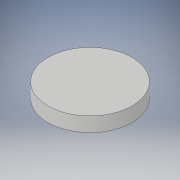
# Autodesk Inventor part: Speaker
Saved by Autodesk Inventor 2018 (Build 220112000, 112)
## iProperties
Created: 2017-05-31
Part Number: Speaker
Material: Generic
Document SubType Name: Modeling
Designer: Rishi
Density: 1 g/cm^3
Appearance: Default
Author: Rishi
Autodesk Inventor part; units mm, degrees
ref_plane "YZ Plane" through (0, 0, 0) normal (1, 0, 0) x (0, 1, 0)
ref_plane "XZ Plane" through (0, 0, 0) normal (0, 1, 0) x (-1, 0, 0)
ref_plane "XY Plane" through (0, 0, 0) normal (0, 0, 1) x (1, 0, 0)
sketch "Sketch1" plane through (0, 0, 0) normal (0, 1, 0) x (-1, 0, 0)
  circle A0 centre (0, 0) radius 14
  dimension "d0" = 28
  constraints: 1 centre point, 1 coincident
  measures "d0" diameter of A0
extrude "Extrusion1" add sketch "Sketch1" along normal blind 4.82
body "Solid1"
